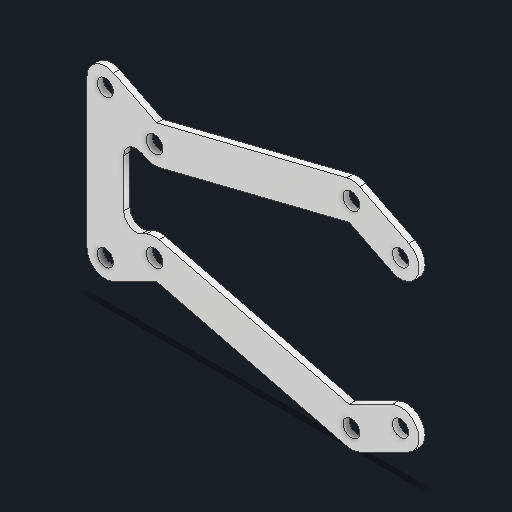
# Autodesk Inventor part: Brain Mount
Saved by Autodesk Inventor 2025.1 (Build 291241000, 241)
## iProperties
Created: 2024-11-19
Part Number: Brain Mount
Material: Acetal Resin, White
Document SubType Name: Modeling
Designer: avere
Density: 1.425 g/cm^3
Appearance: Smooth - White
Author: avere
Autodesk Inventor part; units mm, degrees
ref_plane "YZ Plane" through (0, 0, 0) normal (1, 0, 0) x (0, 1, 0)
ref_plane "XZ Plane" through (0, 0, 0) normal (0, 1, 0) x (-1, 0, 0)
ref_plane "XY Plane" through (0, 0, 0) normal (0, 0, 1) x (1, 0, 0)
sketch "main" plane through (0, 0, 0) normal (0, 0, 1) x (1, 0, 0)
  circle A0 centre (37.6731, -16.4179) radius 2.0955
  circle A1 centre (37.6731, 21.6821) radius 2.0955
  circle A2 centre (24.9731, 28.0321) radius 2.1844
  circle A3 centre (24.9731, -22.7679) radius 2.1844
  circle A4 centre (-38.5364, -16.421) radius 2.0955
  circle A5 centre (-38.5364, 21.679) radius 2.0955
  circle A6 centre (-25.8269, -10.0679) radius 2.1844
  circle A7 centre (-25.8269, 15.3321) radius 2.1844
  arc A8 (-27.9546, 11.0714) -> (-24.6718, 10.7118) centre (-25.8269, 15.3321) ccw
  arc A9 (27.103, 32.2919) -> (23.818, 32.6525) centre (24.9731, 28.0321) ccw
  arc A10 (42.4356, 21.6821) -> (39.803, 25.9419) centre (37.6731, 21.6821) ccw
  arc A11 (39.803, -20.6776) -> (42.4356, -16.4179) centre (37.6731, -16.4179) ccw
  arc A12 (23.818, -27.3882) -> (27.103, -27.0276) centre (24.9731, -22.7679) ccw
  arc A13 (-24.6718, -5.4475) -> (-27.9563, -5.8079) centre (-25.8269, -10.0679) ccw
  arc A14 (-43.2989, -16.421) -> (-36.4069, -20.6809) centre (-38.5364, -16.421) ccw
  arc A15 (-36.4086, 25.9397) -> (-43.2989, 21.679) centre (-38.5364, 21.679) ccw
  line L0 (-43.2989, 21.679) -> (-43.2989, -16.421)
  line L1 (-36.4069, -20.6809) -> (-25.273, -15.1154)
  line L2 (-36.4086, 25.9397) -> (-25.2741, 20.3794)
  line L3 (-25.2741, 20.3794) -> (23.818, 32.6525)
  line L4 (27.103, 32.2919) -> (39.803, 25.9419)
  line L5 (39.803, -20.6776) -> (27.103, -27.0276)
  line L6 (-25.273, -15.1154) -> (23.818, -27.3882)
  line L7 (-27.9546, 11.0714) -> (-29.1804, 11.6835)
  line L8 (-33.7739, 8.843) -> (-33.7739, -3.5793)
  line L9 (-29.1792, -6.4192) -> (-27.9563, -5.8079)
  line L10 (-24.6718, -5.4475) -> (24.419, -17.7203)
  line L11 (24.419, -17.7203) -> (35.5433, -12.1581)
  line L12 (35.5433, 17.4224) -> (24.419, 22.9846)
  line L13 (24.419, 22.9846) -> (-24.6718, 10.7118)
  arc A16 (-33.7739, -3.5793) -> (-29.1792, -6.4192) centre (-30.5989, -3.5793) ccw
  arc A17 (-29.1804, 11.6835) -> (-33.7739, 8.843) centre (-30.5989, 8.843) ccw
  arc A18 (35.5433, 17.4224) -> (39.803, 25.9419) centre (37.6731, 21.6821) ccw
  arc A19 (39.803, -20.6776) -> (35.5433, -12.1581) centre (37.6731, -16.4179) ccw
  point P0 (-0.4291, 2.6313)
  point P1 (-25.8269, -22.7679)
  dimension "d9" = 9.525
  dimension "d10" = 9.525
  dimension "d11" = 9.525
  dimension "d12" = 9.525
  dimension "d13" = 9.525
  dimension "d14" = 9.525
  dimension "d15" = 9.525
  dimension "d16" = 9.525
  dimension "d17" = 9.525
  dimension "d20" = 12.7
  dimension "d21" = 25.4
  dimension "d22" = 3.175
  measures "d9" diameter of A8
  measures "d10" diameter of A9
  measures "d11" diameter of A10
  measures "d12" diameter of A11
  measures "d13" diameter of A12
  measures "d14" diameter of A13
  measures "d15" diameter of A14
  measures "d16" diameter of A15
  measures "d17" distance between parallel lines of L2 L7
  measures "d20" distance of A13.centre point (-25.827, -22.768)
  measures "d21" distance of A13.centre A7.centre
  measures "d22" radius of A16
sketch "Sketch1" plane through (0, 0, 0) normal (0, 0, 1) x (1, 0, 0)
  circle A0 centre (63.5, -6.35) radius 2.0955
  circle A1 centre (63.5, 31.75) radius 2.0955
  circle A2 centre (50.8, 38.1) radius 2.1844
  circle A3 centre (50.8, -12.7) radius 2.1844
  circle A4 centre (-12.7095, -6.3532) radius 2.0955
  circle A5 centre (-12.7095, 31.7468) radius 2.0955
  circle A6 centre (0, 0) radius 2.1844
  circle A7 centre (0, 25.4) radius 2.1844
  arc A8 (-2.1277, 21.1392) -> (1.1551, 20.7797) centre (0, 25.4) ccw
  arc A9 (52.9299, 42.3597) -> (49.6449, 42.7203) centre (50.8, 38.1) ccw
  arc A10 (68.2625, 31.75) -> (65.6299, 36.0097) centre (63.5, 31.75) ccw
  arc A11 (65.6299, -10.6097) -> (68.2625, -6.35) centre (63.5, -6.35) ccw
  arc A12 (49.6449, -17.3203) -> (52.9299, -16.9597) centre (50.8, -12.7) ccw
  arc A13 (1.1551, 4.6203) -> (-2.1294, 4.2599) centre (0, 0) ccw
  arc A14 (-17.472, -6.3532) -> (-10.58, -10.6131) centre (-12.7095, -6.3532) ccw
  arc A15 (-10.5818, 36.0076) -> (-17.472, 31.7468) centre (-12.7095, 31.7468) ccw
  line L0 (-17.472, 31.7468) -> (-17.472, -6.3532)
  line L1 (-10.58, -10.6131) -> (0.5538, -5.0475)
  line L2 (-10.5818, 36.0076) -> (0.5528, 30.4473)
  line L3 (0.5528, 30.4473) -> (49.6449, 42.7203)
  line L4 (52.9299, 42.3597) -> (65.6299, 36.0097)
  line L5 (65.6299, -10.6097) -> (52.9299, -16.9597)
  line L6 (0.5538, -5.0475) -> (49.6449, -17.3203)
  line L7 (-2.1277, 21.1392) -> (-3.3535, 21.7513)
  line L8 (-7.947, 18.9108) -> (-7.947, 6.4886)
  line L9 (-3.3524, 3.6486) -> (-2.1294, 4.2599)
  line L10 (1.1551, 4.6203) -> (50.2459, -7.6524)
  line L11 (50.2459, -7.6524) -> (61.3701, -2.0903)
  line L12 (61.3701, 27.4903) -> (50.2459, 33.0524)
  line L13 (50.2459, 33.0524) -> (1.1551, 20.7797)
  arc A16 (-7.947, 6.4886) -> (-3.3524, 3.6486) centre (-4.772, 6.4886) ccw
  arc A17 (-3.3535, 21.7513) -> (-7.947, 18.9108) centre (-4.772, 18.9108) ccw
  arc A18 (61.3701, 27.4903) -> (65.6299, 36.0097) centre (63.5, 31.75) ccw
  arc A19 (65.6299, -10.6097) -> (61.3701, -2.0903) centre (63.5, -6.35) ccw
  point P0 (68.2625, -6.35)
  point P1 (68.2625, 31.75)
  constraints: 1 other
extrude "Extrusion1" add sketch "Sketch1" along normal blind 1.5875
body "Solid1"
